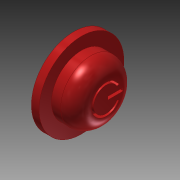
# Autodesk Inventor part: pwr_btn
Saved by Autodesk Inventor 2014 (Build 180170000, 170)
## iProperties
Created: 2017-11-13
Part Number: pwr_btn
Material: Типовые
Document SubType Name: Modeling
Designer: Nikopol
Density: 1 g/cm^3
Appearance: Светло-красный
Author: Nikopol
Autodesk Inventor part; units mm, degrees
ref_plane "YZ Plane" through (0, 0, 0) normal (1, 0, 0) x (0, 1, 0)
ref_plane "XZ Plane" through (0, 0, 0) normal (0, 1, 0) x (-1, 0, 0)
ref_plane "XY Plane" through (0, 0, 0) normal (0, 0, 1) x (1, 0, 0)
sketch "Эскиз1" plane through (0, 0, 0) normal (1, 0, 0) x (0, 1, 0)
  circle A0 centre (0, 0) radius 5.5
  dimension "d0" = 11
  constraints: 1 centre point, 1 coincident
  measures "d0" diameter of A0
extrude "Выдавливание1" add sketch "Эскиз1" along normal blind 1
sketch "Эскиз2" plane through (1, 0, 0) normal (1, 0, 0) x (0, 0, -1)
  circle A0 centre (0, 0) radius 5.5 projected
  circle A1 centre (0, 0) radius 3.9
  dimension "d3" = 7.8
  constraints: 1 centre point, 1 coincident
  measures "d3" diameter of A1
extrude "Выдавливание2" add sketch "Эскиз2" along normal blind 3.2 contours A1
fillet "Сопряжение1" radius 2 1 edges at (4.2, 0, 3.9)
sketch "Эскиз3" plane through (4.2, 0, 0) normal (1, 0, 0) x (0, 0, -1)
  arc A0 (-0.8966, 1.6751) -> (0.9183, 1.6634) centre (0, 0) ccw
  arc A1 (-0.7791, 1.4098) -> (0.7785, 1.4102) centre (0, 0) ccw
  line L0 (-0.7791, 1.4098) -> (-0.8966, 1.6751)
  line L1 (0.7785, 1.4102) -> (0.9183, 1.6634)
  line L2 (-0.2246, 2.2298) -> (0.1754, 2.2298)
  line L3 (0.1754, 2.2298) -> (0.1754, 0.2298)
  line L4 (0.1754, 0.2298) -> (-0.2246, 0.2298)
  line L5 (-0.2246, 0.2298) -> (-0.2246, 2.2298)
  dimension "d9" = 0.4
  dimension "d10" = 2
  constraints: 12 end point, 4 point on circle, 2 centre point, 2 parallel, 1 coincident, 1 horizontal, 1 perpendicular
  measures "d9" distance of L3.end L4.end
  measures "d10" distance of L2.end L3.end
emboss "Рельеф1" sketch "Эскиз3" operation cut depth 1 direction (-1, 0, 0)
